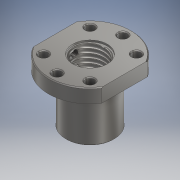
# Autodesk Inventor part: 16mm Lead Nut
Saved by Autodesk Inventor 2018 (Build 220112000, 112)
## iProperties
Created: 2018-03-03
Part Number: 16mm Lead Nut
Material: Stainless Steel, Austenitic
Document SubType Name: Modeling
Designer: Adam
Density: 8 g/cm^3
Appearance: Semi-Polished
Author: Adam
Autodesk Inventor part; units mm, degrees
ref_plane "YZ Plane" through (0, 0, 0) normal (1, 0, 0) x (0, 1, 0)
ref_plane "XZ Plane" through (0, 0, 0) normal (0, 1, 0) x (-1, 0, 0)
ref_plane "XY Plane" through (0, 0, 0) normal (0, 0, 1) x (1, 0, 0)
sketch "Sketch1" plane through (0, 0, 0) normal (0, 0, 1) x (1, 0, 0)
  circle A0 centre (0, 0) radius 11 construction
  line L0 (0, 24) -> (0, -24) construction
  line L1 (-20, 13.2665) -> (-20, -13.2665)
  line L2 (20, 13.2665) -> (20, -13.2665)
  arc A1 (20, 13.2665) -> (-20, 13.2665) centre (0, 0) ccw
  arc A2 (-20, -13.2665) -> (20, -13.2665) centre (0, 0) ccw
  circle A3 centre (0, 0) radius 19 construction
  line L3 (0, 0) -> (13.435, 13.435) construction
  circle A4 centre (13.435, 13.435) radius 2.5
  circle A5 centre (0, 19) radius 2.5
  circle A6 centre (-13.435, 13.435) radius 2.5
  line L4 (0, 0) -> (-20, 0) construction
  circle A7 centre (13.435, -13.435) radius 2.5
  circle A8 centre (0, -19) radius 2.5
  circle A9 centre (-13.435, -13.435) radius 2.5
  line L5 (-17.5, -17.5) -> (17.5, -17.5) construction
  line L6 (17.5, -17.5) -> (17.5, 17.5) construction
  line L7 (17.5, 17.5) -> (-17.5, 17.5) construction
  line L8 (-17.5, 17.5) -> (-17.5, -17.5) construction
  line L9 (-17.5, -17.5) -> (17.5, 17.5) construction
  line L10 (17.5, -17.5) -> (-17.5, 17.5) construction
  dimension "d0" = 22
  dimension "d3" = 20
  dimension "d5" = 24
  dimension "d6" = 38
  dimension "d7" = 45
  dimension "d8" = 5
  dimension "d72" = 35
  dimension "d73" = 35
  constraints: 22 end point, 10 centre point, 8 point on circle, 5 coincident, 4 midpoint, 4 parallel, 4 symmetric about line, 2 equal radius, 1 horizontal, 1 perpendicular, 1 point on line, 1 vertical, 5 other
  measures "d0" diameter of A0
  measures "d3" distance between parallel lines of L2 L0
  measures "d5" radius of A1
  measures "d6" diameter of A3
  measures "d7" angle of L0 L3
  measures "d8" diameter of A4
  measures "d72" distance of L7.end L6.end
  measures "d73" distance of L6.end L5.end
extrude "Extrusion1" add sketch "Sketch1" along normal blind 8
chamfer "Chamfer1" distance 0.5 angle 45 6 edges at (-15.935, 13.435, 8) (-2.5, 19, 8) (10.935, 13.435, 8) (10.935, -13.435, 8) (-2.5, -19, 8) (-15.935, -13.435, 8)
sketch "Sketch2" plane through (0, 0, 0) normal (0, 0, -1) x (-1, 0, 0)
  circle A0 centre (0, 0) radius 14
  dimension "d14" = 28
  constraints: 1 centre point, 1 coincident
  measures "d14" diameter of A0
extrude "Extrusion2" add sketch "Sketch2" along normal blind 28
chamfer "Chamfer2" distance 0.5 angle 45 1 edges at (14, 0, -28)
hole "Hole1" at (0, 0, 8) direction (0, 0, -1) diameter 16 end through all
chamfer "Chamfer3" distance 0.5 angle 45 4 edges at (0, 8, 8) (0, -24, 8) (0, 24, 8) (0, 8, -28)
sketch "Sketch3" plane through (-20, -13.2665, 0) normal (-1, 0, 0) x (0, 0, 1)
  circle A0 centre (3.75, 13.2665) radius 2
  line L0 (0, 26.533) -> (0, 0) projected
  line L1 (0, 0) -> (7.5, 0) projected
  point P0 (0, 13.2665)
  point P1 (0, 13.2665)
  point P2 (3.75, 0)
  dimension "d32" = 4
  constraints: 2 midpoint, 1 centre point, 1 horizontal alignment, 1 vertical alignment
  measures "d32" diameter of A0
extrude "Extrusion3" cut sketch "Sketch3" against normal blind 17
thread "Thread1" size "M4x0.7" class "6H" standard "ANSI Metric M Profile" full length
chamfer "Chamfer4" distance 0.5 angle 45 1 edges at (-20, 0, 1.75)
sketch "Sketch4" plane through (0, 0, 0) normal (1, 0, 0) x (0, 1, 0)
  line L0 (-8.5, 8) -> (-8, 7.5) projected
  line L1 (8.5, 8) -> (8, 7.5) projected
  circle A0 centre (-8, 8) radius 1.394
  circle A1 centre (8, 8) radius 1.394
  line L2 (8.5, 8) -> (-8.5, 8) construction
  line L3 (0, 8) -> (0, 0) construction
  dimension "d44" = 2.788
  constraints: 2 centre point, 2 end point, 1 equal radius, 1 horizontal alignment, 1 midpoint, 1 vertical, 1 vertical alignment, 1 other
  measures "d44" diameter of A0
coil "Coil2" sketch "Sketch4" operation cut axis through (0, 0, 8) along (0, 0, -1) pitch 5 turns 7.2 hand right
sketch "Sketch6" plane through (0, 0, 8) normal (0, 0, 1) x (1, 0, 0)
  circle A0 centre (0, 0) radius 10
  dimension "d66" = 20
  constraints: 1 centre point, 1 coincident
  measures "d66" diameter of A0
extrude "Extrusion5" cut sketch "Sketch6" against normal blind 1
sketch "Sketch7" plane through (0, 0, -28) normal (0, 0, -1) x (-1, 0, 0)
  circle A0 centre (0, 0) radius 10
  dimension "d69" = 20
  constraints: 1 centre point, 1 coincident
  measures "d69" diameter of A0
extrude "Extrusion6" cut sketch "Sketch7" against normal blind 1
body "Solid1"
